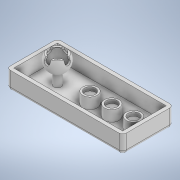
# Autodesk Inventor part: Device Base
Saved by Autodesk Inventor 2021 (Build 250183000, 183)
## iProperties
Created: 2021-03-24
Part Number: Device Base
Material: Generic
Document SubType Name: Modeling
Designer: eng1-127
Density: 1 g/cm^3
Appearance: Default
Author: eng1-127
Autodesk Inventor part; units mm, degrees
ref_plane "YZ Plane" through (0, 0, 0) normal (1, 0, 0) x (0, 1, 0)
ref_plane "XZ Plane" through (0, 0, 0) normal (0, 1, 0) x (-1, 0, 0)
ref_plane "XY Plane" through (0, 0, 0) normal (0, 0, 1) x (1, 0, 0)
sketch "Sketch1" plane through (0, 0, 0) normal (0, 0, 1) x (1, 0, 0)
  arc A0 (0, -12.5) -> (10.3912, 6.9478) centre (0, 0) ccw
  arc A1 (0, -15) -> (12.8118, 7.8012) centre (0, 0) ccw
  line L0 (0, -12.5) -> (0, -15)
  line L1 (0, -15) -> (0, -30)
  line L2 (0, -30) -> (5.0613, -30)
  line L3 (5.0613, -30) -> (5.0613, -14.1203)
  line L4 (12.8118, 7.8012) -> (10.3912, 7.8012)
  line L5 (10.3912, 6.9478) -> (10.3912, 7.8012)
  dimension "d0" = 25
  dimension "d2" = 30
  dimension "d3" = 15
  constraints: 12 end point, 5 point on circle, 2 centre point, 2 coincident, 2 perpendicular, 2 vertical, 1 horizontal
  measures "d0" diameter of A0
  measures "d2" diameter of A1
  measures "d3" distance of L0.end L1.end
revolve "Revolution1" add sketch "Sketch1" angle 360 about axis through (0, -15, 0) along (0, -1, 0)
sketch "Sketch2" plane through (0, 7.8012, 0) normal (0, 1, 0) x (1, 0, 0)
  line L0 (0.0071, 24.1346) -> (3.7571, 24.1346)
  line L1 (3.7571, 24.1346) -> (3.7571, -20.7692)
  line L2 (3.7571, -20.7692) -> (0.0071, -20.7692)
  line L3 (0.0071, -20.7692) -> (0.0071, 24.1346)
  line L4 (0.0071, 21.7767) -> (-3.7429, 21.7767)
  line L5 (-3.7429, 21.7767) -> (-3.7429, -17.1832)
  line L6 (-3.7429, -17.1832) -> (0.0071, -17.1832)
  line L7 (0.0071, -17.1832) -> (0.0071, 21.7767)
  line L8 (-20.2456, 0) -> (19.1397, 0)
  line L9 (19.1397, 0) -> (19.1397, 3.75)
  line L10 (19.1397, 3.75) -> (-20.2456, 3.75)
  line L11 (-20.2456, 3.75) -> (-20.2456, 0)
  line L12 (-17.6085, 0) -> (17.6085, 0)
  line L13 (17.6085, 0) -> (17.6085, -3.75)
  line L14 (17.6085, -3.75) -> (-17.6085, -3.75)
  line L15 (-17.6085, -3.75) -> (-17.6085, 0)
  point P0 (0, 0)
  point P1 (-3.7429, -3.75)
  point P2 (-3.7429, 3.75)
  point P3 (3.7571, 3.75)
  point P4 (3.7571, -3.75)
  point P5 (17.6085, 0)
  point P6 (0.0071, -17.1832)
  dimension "d5" = 3.75
  dimension "d6" = 3.75
  dimension "d7" = 3.75
  dimension "d8" = 3.75
  constraints: 32 end point, 8 parallel, 4 horizontal, 4 perpendicular, 2 point on line
  measures "d5" distance of L0.start L0.end
  measures "d6" distance of L4.start L4.end
  measures "d7" distance of L8.end L9.end
  measures "d8" distance of L14.end L12.start
extrude "Extrusion1" cut sketch "Sketch2" against normal blind 7.5 contours L0 L1 L10 L3 | L3 L10 L5 L4 | L10 L9 L8 L1 | L8 L13 L14 L1 | L5 L8 L11 L10 | L1 L2 L3 L14 | L3 L6 L5 L14 | L5 L14 L15 L8
fillet "Fillet1" radius 3.75 8 edges at (-3.7429, 0.3012, 13.2225) (-3.7429, 0.3012, -13.2225) (13.2205, 0.3012, -3.75) (-13.2205, 0.3012, -3.75) (3.7571, 0.3012, 13.2185) (3.7571, 0.3012, -13.2185) (13.2205, 0.3012, 3.75) (-13.2205, 0.3012, 3.75)
sketch "Sketch3" plane through (0, -30, 0) normal (0, -1, 0) x (1, 0, 0)
  line L0 (0, 0) -> (-30, 0)
  line L1 (-30, 0) -> (-30, 30)
  line L2 (-30, 30) -> (0, 30)
  line L3 (0, 30) -> (0, 0)
  circle A0 centre (0, 0) radius 5.0613 projected
  line L4 (0, 0) -> (-30, 0)
  line L5 (-30, 0) -> (-30, -30)
  line L6 (-30, -30) -> (0, -30)
  line L7 (0, -30) -> (0, 0)
  line L8 (0, 30) -> (120, 30)
  line L9 (120, 30) -> (120, -30)
  line L10 (120, -30) -> (0, -30)
  line L11 (0, -30) -> (0, 30)
  dimension "d12" = 30
  dimension "d13" = 30
  dimension "d14" = 30
  dimension "d15" = 120
  constraints: 24 end point, 6 parallel, 3 horizontal, 3 perpendicular
  measures "d12" distance of L0.end L1.end
  measures "d13" distance of L1.end L2.end
  measures "d14" distance of L4.end L5.end
  measures "d15" distance of L9.end L10.end
extrude "Extrusion2" add sketch "Sketch3" along normal blind 5
sketch "Sketch4" plane through (-30, -30, -30) normal (-1, 0, 0) x (0, 0, 1)
  line L0 (0, -5) -> (60, -5)
  line L1 (60, -5) -> (60, 20)
  line L2 (60, 20) -> (0, 20)
  line L3 (0, 20) -> (0, -5)
  point P0 (30, 30)
  dimension "d18" = 60
  dimension "d19" = 25
  constraints: 8 end point, 2 parallel, 1 horizontal, 1 perpendicular
  measures "d18" distance of L0.start L0.end
  measures "d19" distance of L0.end L1.end
extrude "Extrusion3" add sketch "Sketch4" along normal blind 5
sketch "Sketch5" plane through (120, -35, -30) normal (0, 0, -1) x (-1, 0, 0)
  line L0 (155, 25) -> (155, 0) projected
  line L1 (0, 0) -> (155, 0) projected
  line L2 (155, 25) -> (0, 25)
  line L3 (0, 25) -> (0, 0)
  line L4 (0, 0) -> (155, 0)
  line L5 (155, 0) -> (155, 25)
  point P0 (120, 35)
  constraints: 8 end point, 2 parallel, 1 horizontal, 1 perpendicular
extrude "Extrusion4" add sketch "Sketch5" along normal blind 5
sketch "Sketch6" plane through (120, -35, 30) normal (1, 0, 0) x (0, 0, -1)
  line L0 (0, 25) -> (65, 25) projected
  line L1 (0, 0) -> (65, 0) projected
  line L2 (65, 25) -> (0, 25)
  line L3 (0, 25) -> (0, 0)
  line L4 (0, 0) -> (65, 0)
  line L5 (65, 0) -> (65, 25)
  point P0 (30, 35)
  constraints: 8 end point, 2 parallel, 1 horizontal, 1 perpendicular
extrude "Extrusion5" add sketch "Sketch6" along normal blind 5
sketch "Sketch7" plane through (0, -30, 0) normal (0, 1, 0) x (1, 0, 0)
  line L0 (-30, 30) -> (120, 30) projected
  line L1 (120, 30) -> (90, 30)
  line L2 (90, 30) -> (90, -30)
  line L3 (90, -30) -> (120, -30)
  line L4 (120, -30) -> (120, 30)
  line L5 (90, 30) -> (60, 30)
  line L6 (60, 30) -> (60, -30)
  line L7 (60, -30) -> (90, -30)
  line L8 (90, -30) -> (90, 30)
  line L9 (60, 30) -> (30, 30)
  line L10 (30, 30) -> (30, -30)
  line L11 (30, -30) -> (60, -30)
  line L12 (60, -30) -> (60, 30)
  circle A0 centre (45, 0) radius 10
  circle A1 centre (75, 0) radius 10
  circle A2 centre (105, 0) radius 10
  point P0 (0, 0)
  dimension "d27" = 30
  dimension "d29" = 30
  dimension "d30" = 30
  dimension "d31" = 60
  dimension "d32" = 20
  constraints: 24 end point, 6 parallel, 3 centre point, 3 horizontal, 3 perpendicular
  measures "d27" distance of L2.end L3.end
  measures "d29" distance of L6.end L7.end
  measures "d30" distance of L10.end L11.end
  measures "d31" distance of L9.end L10.end
  measures "d32" diameter of A0
extrude "Extrusion6" add sketch "Sketch7" along normal blind 15 contours A0 | A1 | A2
sketch "Sketch8" plane through (45, -15, 0) normal (0, 1, 0) x (1, 0, 0)
  circle A0 centre (0, 0) radius 7.5
  circle A1 centre (30, 0) radius 10 projected
  circle A2 centre (30, 0) radius 7.5
  circle A3 centre (60, 0) radius 10 projected
  circle A4 centre (60, 0) radius 7.5
  point P0 (-45, 0)
  dimension "d35" = 15
  constraints: 3 centre point, 2 coincident
  measures "d35" diameter of A0
extrude "Extrusion7" cut sketch "Sketch8" against normal blind 5 contours A0 | A2 | A4
sketch "Sketch9" plane through (-30, -30, 30) normal (0, 0, 1) x (1, 0, 0)
  line L0 (-5, -5) -> (155, -5) projected
  line L1 (155, 20) -> (155, -5) projected
  line L2 (-5, -5) -> (155, -5)
  line L3 (155, -5) -> (155, 20)
  line L4 (155, 20) -> (-5, 20)
  line L5 (-5, 20) -> (-5, -5)
  point P0 (30, 30)
  constraints: 8 end point, 2 parallel, 1 horizontal, 1 perpendicular
extrude "Extrusion8" add sketch "Sketch9" along normal blind 5
fillet "Fillet2" radius 5 8 edges at (45, -35, 35) (125, -22.5, 35) (-35, -22.5, 35) (-35, -22.5, -35) (-35, -35, 0) (45, -35, -35) (125, -35, 0) (125, -22.5, -35)
body "Solid1"
